mj_sign_holder (Autodesk Fusion 360 design; units mm, degrees)
Autodesk Fusion 360 part; units mm, degrees
sketch "Sketch1" plane through (0, 0, 0) normal (0, 1, 0) x (1, 0, 0)
  circle A0 centre (0, 0) radius 1.5
  circle A1 centre (165, 0) radius 1.5
  circle A2 centre (0, 265) radius 1.5
  circle A3 centre (165, 265) radius 1.5
  line L0 (0, 0) -> (0, 265) construction
  line L1 (0, 0) -> (165, 0) construction
  line L2 (165, 0) -> (165, 265) construction
  line L3 (165, 265) -> (0, 265) construction
  circle A4 centre (0, 0) radius 6
  circle A5 centre (165, 0) radius 6
  circle A6 centre (165, 265) radius 6
  circle A7 centre (0, 265) radius 6
  line L4 (-5.0934, 261.8286) -> (159.9066, -3.1714)
  line L5 (5.0934, 268.1714) -> (170.0934, 3.1714)
  line L6 (5.0934, -3.1714) -> (170.0934, 261.8286)
  line L7 (159.9066, 268.1714) -> (-5.0934, 3.1714)
  line L8 (0, -6) -> (165, -6)
  line L9 (165, 6) -> (0, 6)
  line L10 (165, 271) -> (0, 271)
  line L11 (0, 259) -> (165, 259)
  line L12 (72.5, 105.0878) -> (92.5, 105.0878)
  line L13 (72.5, 159.9122) -> (92.5, 159.9122)
  circle A8 centre (82.5, 115.1484) radius 1
  circle A9 centre (82.5, 149.8516) radius 1
  line L14 (82.5, 149.8516) -> (82.5, 115.1484) construction
  point P0 (82.5, 143.8516)
  point P1 (82.5, 121.1484)
  dimension "d1" = 165
  dimension "d2" = 265
  dimension "d3" = 3
  dimension "d4" = 3
  dimension "d5" = 3
  dimension "d6" = 3
  dimension "d7" = 12
  dimension "d8" = 12
  dimension "d9" = 12
  dimension "d10" = 12
  dimension "d11" = 20
  dimension "d12" = 20
  dimension "d13" = 2
  dimension "d14" = 2
  dimension "d15" = 6
  dimension "d16" = 6
  constraint coincident A0.centre L0.start
  constraint coincident A2.centre L0.end
  constraint vertical L0
  constraint coincident A1.centre L1.end
  constraint perpendicular L0 L1
  constraint coincident A3.centre L2.end
  constraint perpendicular L1 L2
  constraint horizontal L3
  constraint concentric A0 A4
  constraint concentric A1 A5
  constraint concentric A3 A6
  constraint concentric A2 A7
  constraint coincident A7 L4.start
  constraint coincident A5 L4.end
  constraint tangent A5 L4
  constraint tangent A7 L4
  constraint coincident A7 L5.start
  constraint coincident A5 L5.end
  constraint tangent A5 L5
  constraint coincident A4 L6.start
  constraint coincident A6 L6.end
  constraint tangent A6 L6
  constraint coincident A6 L7.start
  constraint coincident A4 L7.end
  constraint tangent A4 L7
  constraint tangent A6 L7
  constraint tangent A7 L5
  constraint tangent A4 L6
  constraint coincident A4 L8.start
  constraint coincident A5 L8.end
  constraint tangent A5 L8
  constraint horizontal L8
  constraint coincident A5 L9.start
  constraint coincident L2 L9.start
  constraint coincident L0 L9.end
  constraint coincident A4 L9.end
  constraint coincident A6 L10.start
  constraint coincident A7 L10.end
  constraint tangent A7 L10
  constraint horizontal L10
  constraint coincident A7 L11.start
  constraint coincident L0 L11.start
  constraint coincident A6 L11.end
  constraint coincident L2 L11.end
  constraint coincident L6 L12.start
  constraint coincident L4 L12.end
  constraint horizontal L12
  constraint coincident L5 L13.start
  constraint coincident L7 L13.end
  constraint parallel L12 L13
  constraint coincident A9.centre L14.start
  constraint coincident A8.centre L14.end
  constraint vertical L14
  constraint coincident L7 P0
  constraint coincident L5 P0
  constraint coincident L14 P0
  constraint coincident L14 P1
  constraint coincident L4 P1
  measures "d1" distance of A0.centre A1.centre
  measures "d2" distance of A0.centre A2.centre
  measures "d3" diameter of A0
  measures "d4" diameter of A1
  measures "d5" diameter of A3
  measures "d6" diameter of A2
  measures "d7" diameter of A4
  measures "d8" diameter of A5
  measures "d9" diameter of A6
  measures "d10" diameter of A7
  measures "d11" distance of L12.start L12.end
  measures "d12" distance of L13.start L13.end
  measures "d13" diameter of A9
  measures "d14" diameter of A8
  measures "d15" distance of A8.centre P1
  measures "d16" distance of A9.centre P0
extrude "Extrude1" add sketch "Sketch1" along normal blind 8 contours A4 | A4 L6 L9 | A4 L4 L6 L7 L9 | A4 A5 L4 L6 L8 L9 | L4 L5 L6 L7 | A7 L4 L5 L7 L11 | L4 L6 L12 | A5 L4 L9 | A5 L4 L5 L6 L9 | A5 | A7 | A6 L5 L6 L7 L11 | L5 L7 L13 | A6 A7 L5 L7 L10 L11 | A7 L5 L11 | A6 | A6 L7 L11
equation "d4 = d3"
equation "d5 = d3"
equation "d6 = d3"
equation "d8 = d7"
equation "d9 = d7"
equation "d10 = d7"
equation "d12 = d11"
equation "d14 = d13"
equation "d16 = d15"
